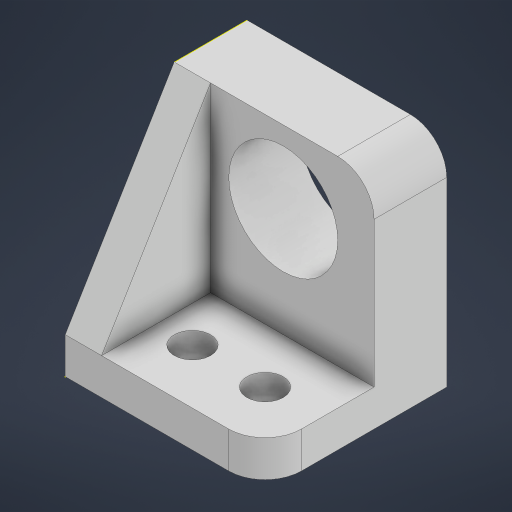
# Autodesk Inventor part: Część15
Saved by Autodesk Inventor 2023 (Build 270158000, 158)
## iProperties
Created: 2023-05-08
Part Number: Część15
Material: Ogólny
Document SubType Name: Modeling
Designer: Adam
Density: 1 g/cm^3
Appearance: Domyślna
Author: Adam
Autodesk Inventor part; units mm, degrees
ref_plane "YZ Plane" through (0, 0, 0) normal (1, 0, 0) x (0, 1, 0)
ref_plane "XZ Plane" through (0, 0, 0) normal (0, 1, 0) x (-1, 0, 0)
ref_plane "XY Plane" through (0, 0, 0) normal (0, 0, 1) x (1, 0, 0)
sketch "Szkic1" plane through (0, 0, 0) normal (0, 1, 0) x (-1, 0, 0)
  line L0 (0, 0) -> (-45, 0)
  line L1 (-55, -10) -> (-55, -50)
  line L2 (-55, -50) -> (0, -50)
  line L3 (0, -50) -> (0, 0)
  arc A0 (-45, 0) -> (-55, -10) centre (-45, -10) ccw
  point P0 (-55, 0)
  dimension "d0" = 55
  dimension "d1" = 50
  dimension "d2" = 10
  constraints: 8 end point, 2 parallel, 2 point on circle, 2 point on line, 2 tangent, 1 centre point, 1 horizontal, 1 perpendicular
  measures "d0" distance of L2.end L1.end
  measures "d1" distance of L1.end point (-55, 0)
  measures "d2" radius of A0
extrude "Wyciągnięcie proste1" add sketch "Szkic1" along normal blind 10
sketch "Szkic2" plane through (0, 10, 0) normal (0, 1, 0) x (1, 0, 0)
  line L0 (0, 50) -> (0, 0) projected
  line L1 (0, 50) -> (55, 50)
  line L2 (55, 50) -> (55, 30)
  line L3 (55, 30) -> (0, 30)
  line L4 (0, 30) -> (0, 50)
  dimension "d5" = 55
  dimension "d6" = 20
  constraints: 8 end point, 2 parallel, 1 horizontal, 1 perpendicular
  measures "d5" distance of L2.end L3.end
  measures "d6" distance of L1.end L2.end
extrude "Wyciągnięcie proste2" add sketch "Szkic2" along normal blind 50
fillet "Zaokrąglenie1" radius 10 1 edges at (55, 60, -40)
sketch "Szkic3" plane through (0, 0, 0) normal (1, 0, 0) x (0, 1, 0)
  line L0 (0, -50) -> (0, 0) projected
  line L1 (0, 0) -> (10, 0) projected
  line L2 (10, -30) -> (10, 0) projected
  line L3 (10, -30) -> (60, -30) projected
  line L4 (60, -50) -> (60, -30) projected
  line L5 (0, -50) -> (60, -50) projected
  line L6 (60, -30) -> (50, -30) projected
  line L7 (10, -30) -> (60, -30) projected
  line L8 (10, -30) -> (50, -30) projected
  line L9 (60, -30) -> (10, 0)
  constraints: 2 end point, 1 other
sketch "Szkic4" plane through (0, 0, 0) normal (1, 0, 0) x (0, 1, 0)
  line L0 (60, -50) -> (60, -30) projected
  line L1 (10, -30) -> (50, -30) projected
  line L2 (60, -30) -> (10, -30)
  line L3 (10, -10) -> (10, 0) projected
  line L4 (10, -30) -> (10, 0)
  point P0 (0, 0)
  constraints: 4 end point, 1 collinear, 1 perpendicular
extrude "Wyciągnięcie proste3" add sketch "Szkic3" along normal blind 10 contours L9 L3 L2
sketch "Szkic5" plane through (55, 10, -30) normal (0, 0, 1) x (1, 0, 0)
  line L0 (0, 0) -> (0, 40) projected
  line L1 (-45, 0) -> (-10, 0) projected
  point P0 (-55, -10)
  point P1 (-25, 30)
  dimension "d12" = 25
  dimension "d13" = 30
  measures "d12" distance from line of L0 point (-25, 30)
  measures "d13" distance from line of L1 point (-25, 30)
hole "Otwór1" at (30, 40, -30) direction (0, 0, -1) diameter 30 end through all
sketch "Szkic6" plane through (0, 10, 0) normal (0, 1, 0) x (1, 0, 0)
  line L0 (10, 30) -> (10, 0) projected
  line L1 (10, 30) -> (45, 30) projected
  point P0 (0, 0)
  point P1 (40, 15)
  point P2 (20, 15)
  dimension "d21" = 10
  dimension "d22" = 20
  dimension "d23" = 15
  measures "d21" distance from line of point (20, 15) L0
  measures "d22" distance of point (40, 15) point (20, 15)
  measures "d23" distance from line of L1 point (40, 15)
hole "Otwór2" at (20, 10, -15) at (40, 10, -15) direction (0, -1, 0) diameter 10 end through all
